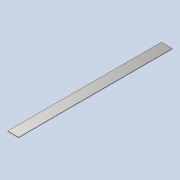
# Autodesk Inventor part: tasiemka_do_zgrzewania_2
Saved by Autodesk Inventor 2021.3 (Build 253353000, 353)
## iProperties
Created: 2023-05-23
Part Number: tasiemka_do_zgrzewania_2
Material: Ogólny
Document SubType Name: Modeling
Designer: User
Density: 1 g/cm^3
Appearance: Nierdzewna — szczotkowana
Author: User
Autodesk Inventor part; units mm, degrees
ref_plane "YZ Plane" through (0, 0, 0) normal (1, 0, 0) x (0, 1, 0)
ref_plane "XZ Plane" through (0, 0, 0) normal (0, 1, 0) x (-1, 0, 0)
ref_plane "XY Plane" through (0, 0, 0) normal (0, 0, 1) x (1, 0, 0)
sketch "Szkic1" plane through (0, 0, 0) normal (0, 1, 0) x (-1, 0, 0)
  line L0 (31.5094, 1014.1509) -> (-38.4906, 1014.1509)
  line L1 (-38.4906, 1014.1509) -> (-38.4906, 24.1509)
  line L2 (-38.4906, 24.1509) -> (31.5094, 24.1509)
  line L3 (31.5094, 24.1509) -> (31.5094, 1014.1509)
  point P0 (0, 0)
  dimension "d0" = 70
  dimension "d1" = 990
  constraints: 8 end point, 2 parallel, 1 horizontal, 1 perpendicular
  measures "d0" distance between parallel lines of L1 L3
  measures "d1" distance of L2.end L0.start
extrude "Wyciągnięcie proste1" add sketch "Szkic1" along normal blind 3
